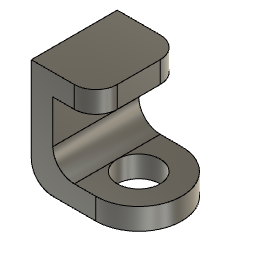
Exercie_3 (Autodesk Fusion 360 design; units mm, degrees)
Autodesk Fusion 360 part; units mm, degrees
sketch "Sketch1" plane through (0, 0, 0) normal (0, 0, 1) x (1, 0, 0)
  line L0 (0, 0) -> (30, 0)
  line L1 (30, 0) -> (30, 40)
  line L2 (30, 40) -> (0, 40)
  line L3 (0, 40) -> (0, 0)
  arc A0 (30, 0) -> (30, 40) centre (30, 20) ccw
  dimension "d1" = 30
  dimension "d2" = 40
  dimension "d3" = 40
  constraint horizontal L0
  constraint vertical L1
  constraint horizontal L2
  constraint vertical L3
  constraint coincident L0.start L3.end
  measures "d1" distance of L0.start L0.end
  measures "d2" distance of L0.start L2.end
  measures "d3" diameter of A0
extrude "Extrude1" add sketch "Sketch1" along normal blind 10
sketch "Sketch2" plane through (0, 0, 10) normal (0, 0, 1) x (-1, 0, 0)
  arc A0 (-30, 0) -> (-30, -40) centre (-30, -20) ccw
  line L0 (-30, -40) -> (0, -40)
  line L1 (0, -40) -> (0, 0)
  line L2 (0, 0) -> (-30, 0)
  line L3 (0, -40) -> (-10, -40)
  line L4 (-10, -40) -> (-10, 0)
  line L5 (-10, 0) -> (0, 0)
  line L6 (0, 0) -> (0, -40)
  dimension "d6" = 10
  dimension "d7" = 40
  constraint horizontal L3
  constraint vertical L4
  constraint horizontal L5
  constraint vertical L6
  constraint coincident L1.end L2.start
  measures "d6" distance of L0.end L3.end
  measures "d7" distance of L3.end L4.end
extrude "Extrude2" add sketch "Sketch2" along normal blind 30.06 contours L0 L1 L2 L3 L4 L5 L6
sketch "Sketch3" plane through (0, 0, 40.06) normal (0, 0, 1) x (-1, 0, 0)
  line L0 (0, 0) -> (-10, 0)
  line L1 (-10, 0) -> (-10, -40)
  line L2 (-10, -40) -> (0, -40)
  line L3 (0, -40) -> (0, 0)
  line L4 (0, -40) -> (-30, -40)
  line L5 (-30, -40) -> (-30, 0)
  line L6 (-30, 0) -> (0, 0)
  line L7 (0, 0) -> (0, -40)
  dimension "d10" = 30
  dimension "d11" = 40
  constraint horizontal L4
  constraint vertical L5
  constraint horizontal L6
  constraint vertical L7
  constraint coincident L0.start L3.end
  measures "d10" distance of L2.end L4.end
  measures "d11" distance of L4.end L5.end
extrude "Extrude3" add sketch "Sketch3" along normal blind 10
fillet "Fillet1" radius 10 4 edges at (30, 0, 45.06) (30, 40, 45.06) (10, 20, 10) (0, 20, 0)
hole "Hole1" at (30, 20, 10) direction (0, 0, -1) diameter 20 end through all
